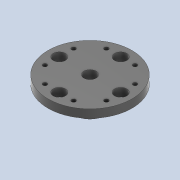
# Autodesk Inventor part: ServoHorn_Circle
Saved by Autodesk Inventor 2021.2 (Build 252289000, 289)
## iProperties
Created: 2021-03-29
Part Number: ServoHorn_Circle
Material: ABS プラスチック
Document SubType Name: Modeling
Designer: Hagihara Yuya
Density: 1.06 g/cm^3
Appearance: 滑らか - 黒
Author: Hagihara Yuya
Autodesk Inventor part; units mm, degrees
ref_plane "YZ Plane" through (0, 0, 0) normal (1, 0, 0) x (0, 1, 0)
ref_plane "XZ Plane" through (0, 0, 0) normal (0, 1, 0) x (-1, 0, 0)
ref_plane "XY Plane" through (0, 0, 0) normal (0, 0, 1) x (1, 0, 0)
sketch "スケッチ1" plane through (0, 0, 0) normal (0, 0, 1) x (1, 0, 0)
  circle A0 centre (0, 0) radius 10.25
  dimension "d0" = 20.5
  constraints: 1 centre point, 1 coincident
  measures "d0" diameter of A0
extrude "押し出し1" add sketch "スケッチ1" along normal blind 2
sketch "スケッチ2" plane through (0, 0, 0) normal (0, 0, -1) x (-1, 0, 0)
  circle A0 centre (0, 0) radius 4.1
  dimension "d3" = 8.2
  constraints: 1 centre point, 1 coincident
  measures "d3" diameter of A0
extrude "押し出し2" add sketch "スケッチ2" along normal blind 4.5
sketch "スケッチ3" plane through (0, 0, -4.5) normal (0, 0, -1) x (-1, 0, 0)
  point P0 (0, 0)
  point P1 (0, 0)
  constraints: 1 coincident
hole "穴1" at (0, 0, -4.5) direction (0, 0, 1) diameter 3 end through all counterbore diameter 6 counterbore depth 4
sketch "スケッチ4" plane through (0, 0, 2) normal (0, 0, 1) x (1, 0, 0)
  point P0 (0, 0)
  point P1 (7.5, 0)
  point P2 (0, 7.5)
  point P3 (-7.5, 0)
  point P4 (0, -7.5)
  dimension "d13" = 7.5
  dimension "d16" = 360
  constraints: 1 horizontal alignment, 5 other
  measures "d13" distance of point (0, 0) point (7.5, 0)
hole "穴2" at (7.5, 0, 2) at (0, 7.5, 2) at (-7.5, 0, 2) at (0, -7.5, 2) direction (0, 0, -1) diameter 3 end through all
sketch "スケッチ5" plane through (0, 0, 2) normal (0, 0, 1) x (1, 0, 0)
  circle A0 centre (7.5, 0) radius 1.5 projected
  point P0 (0, 0)
  point P1 (7.5, 3.5)
  point P2 (7.5, -3.5)
  point P3 (-3.5, 7.5)
  point P4 (3.5, 7.5)
  point P5 (-7.5, -3.5)
  point P6 (-7.5, 3.5)
  point P7 (3.5, -7.5)
  point P8 (-3.5, -7.5)
  dimension "d25" = 3.5
  dimension "d26" = 3.5
  dimension "d29" = 360
  constraints: 2 vertical alignment, 9 other
  measures "d25" distance of A0.centre point (7.5, -3.5)
  measures "d26" distance of point (7.5, 3.5) A0.centre
hole "穴3" at (7.5, 3.5, 2) at (7.5, -3.5, 2) at (-3.5, 7.5, 2) at (3.5, 7.5, 2) at (-7.5, -3.5, 2) at (-7.5, 3.5, 2) at (3.5, -7.5, 2) at (-3.5, -7.5, 2) direction (0, 0, -1) diameter 1 end through all
equation "\"d26\" = d25"
